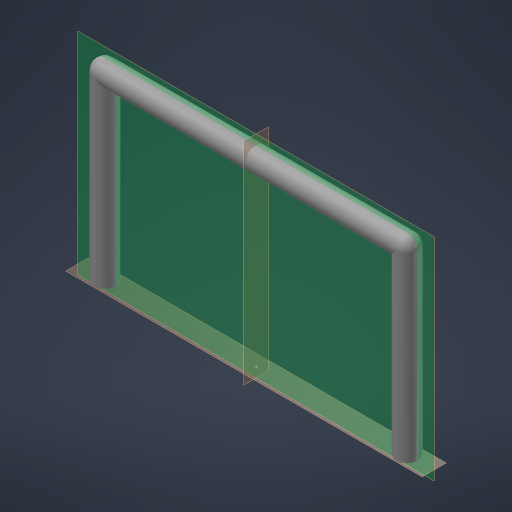
# Autodesk Inventor part: Wire
Saved by Autodesk Inventor 2024 (Build 280153000, 153)
## iProperties
Created: 2023-12-28
Part Number: Wire
Material: S235
Catalog Web Link: http://emmausbovenbouw.op-weg.be/
Vendor: Emmaüsinstituut Bovenbouw Aalter
Document SubType Name: Modeling
Designer: Louis
Engineer: Declercq St.
Manufacturer: Standard
Standards Organization: Custom
Density: 7.86 g/cm^3
Appearance: Steel
Manager: Louis Van Roosmaelen
Company: DCS - DIGITAL COMBAT SIMULATOR
Title: F18C Home Cockpit
Author: Louis
Keywords: Ø
IDENT.NR.: AJ2022
TEAM: 30
Autodesk Inventor part; units mm, degrees
sketch "Sketch1" plane through (0, 0, 0) normal (0, 0, 1) x (1, 0, 0)
  circle A0 centre (-5, 0) radius 0.3635
  circle A1 centre (5, 0) radius 0.3635
  line L0 (-7.5089, 0) -> (7.5089, 0) projected
  point P0 (0, 0)
  point P1 (-5.3635, 0)
  point P2 (-4.6365, 0)
  dimension "d2" = 0.727
  dimension "d3" = 0.727
  dimension "d4" = 10
  dimension "d5" = 5
  constraints: 2 centre point, 2 point on line
  measures "d2" diameter of A0
  measures "d3" diameter of A1
  measures "d4" distance of A0.centre A1.centre
  measures "d5" distance of point (0, 0) A0.centre
extrude "Extrusion1" add sketch "Sketch1" along normal blind 6
sketch "Sketch2" plane through (0, 0, 0) normal (0, 1, 0) x (-1, 0, 0)
  line L0 (-4.6365, 6) -> (-5.3635, 6) projected
  circle A0 centre (-5, 6) radius 0.3635
  line L1 (5.3635, 6) -> (4.6365, 6) projected
  circle A1 centre (5, 6) radius 0.3635
  line L2 (5, 6.3635) -> (-5, 6.3635)
  line L3 (-5, 6) -> (5, 6)
  point P0 (0, 0)
  constraints: 4 end point, 4 point on circle, 2 centre point, 2 midpoint, 2 tangent, 1 collinear
revolve "Revolution1" add sketch "Sketch2" angle 360 about axis through (5, 0, 6) along (-1, 0, 0) picked at (-5.1703, 6.1703) picked at (4.8297, 6.1703) contours L0 A0 | A0 L2 A1 L3 | A1 L1
equation "\"d5\" = 0.5 * d4"
body "Solid1"
